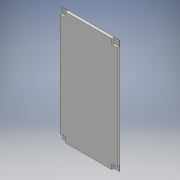
# Autodesk Inventor part: BODY_TOP_COVER
Saved by Autodesk Inventor 2017 (Build 210142000, 142)
## iProperties
Created: 2018-01-04
Part Number: BODY_TOP_COVER
Material: Generic
Document SubType Name: Modeling
Designer: Alex
Density: 1 g/cm^3
Appearance: Default
Author: Alex
Autodesk Inventor part; units mm, degrees
ref_plane "YZ Plane" through (0, 0, 0) normal (1, 0, 0) x (0, 1, 0)
ref_plane "XZ Plane" through (0, 0, 0) normal (0, 1, 0) x (-1, 0, 0)
ref_plane "XY Plane" through (0, 0, 0) normal (0, 0, 1) x (1, 0, 0)
sketch "Sketch1" plane through (0, 0, 0) normal (0, 1, 0) x (-1, 0, 0)
  line L0 (-27.5, 55) -> (27.5, 55)
  line L1 (27.5, 55) -> (27.5, -55)
  line L2 (27.5, -55) -> (-27.5, -55)
  line L3 (-27.5, -55) -> (-27.5, 55)
  point P0 (0, 0)
  point P1 (0, -55)
  point P2 (27.5, 0)
  dimension "d0" = 110
  dimension "d1" = 55
  constraints: 8 end point, 2 midpoint, 2 parallel, 1 horizontal, 1 horizontal alignment, 1 perpendicular, 1 vertical alignment
  measures "d0" distance of L0.end L1.end
  measures "d1" distance of L0.start L0.end
extrude "Extrusion1" add sketch "Sketch1" along normal blind 2.5
sketch "Sketch2" plane through (0, 0, 0) normal (0, -1, 0) x (1, 0, 0)
  line L0 (27.5, 50) -> (22.5, 50)
  line L1 (22.5, 50) -> (22.5, 55)
  line L2 (22.5, 55) -> (27.5, 55)
  line L3 (27.5, 55) -> (27.5, 50)
  line L4 (27.5, -55) -> (27.5, 55) projected
  line L5 (27.5, 55) -> (-27.5, 55) projected
  line L6 (0, -77) -> (0, 77) projected
  line L7 (-38.5, 0) -> (38.5, 0) projected
  line L8 (27.5, -50) -> (22.5, -50)
  line L9 (22.5, -50) -> (22.5, -55)
  line L10 (22.5, -55) -> (27.5, -55)
  line L11 (27.5, -55) -> (27.5, -50)
  line L12 (-27.5, 50) -> (-22.5, 50)
  line L13 (-22.5, 50) -> (-22.5, 55)
  line L14 (-22.5, 55) -> (-27.5, 55)
  line L15 (-27.5, 55) -> (-27.5, 50)
  line L16 (-22.5, -50) -> (-22.5, -55)
  line L17 (-27.5, -50) -> (-22.5, -50)
  line L18 (-27.5, -55) -> (-27.5, -50)
  line L19 (-22.5, -55) -> (-27.5, -55)
  point P0 (0, 0)
  dimension "d4" = 5
  constraints: 32 end point, 12 symmetric about line, 2 collinear, 2 parallel, 2 perpendicular, 1 horizontal
  measures "d4" distance of L0.start L0.end
extrude "Extrusion2" cut sketch "Sketch2" against normal blind 2 contours L0 L1 L2 L3 | L10 L9 L8 L4 | L13 L12 L15 L5 | L16 L19 L18 L17
equation "\"d2\" = 0.5 * body_C_Top"
equation "\"d4\" = magnet_A"
equation "\"d5\" = magnet_B"
equation "\"body_C_Top\" = 5"
equation "\"magnet_A\" = 5"
equation "\"magnet_B\" = 2"
body "Solid1"
